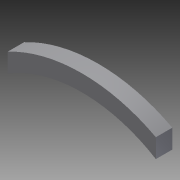
# Autodesk Inventor part: motor stay top
Saved by Autodesk Inventor 2012 (Build 160160000, 160)
## iProperties
Created: 2012-02-05
Part Number: motor stay top
Material: Default
Document SubType Name: Modeling
Designer: Antonella Wilby
Density: 1 g/cm^3
Author: Antonella Wilby
Autodesk Inventor part; units mm, degrees
ref_plane "YZ Plane" through (0, 0, 0) normal (1, 0, 0) x (0, 1, 0)
ref_plane "XZ Plane" through (0, 0, 0) normal (0, 1, 0) x (-1, 0, 0)
ref_plane "XY Plane" through (0, 0, 0) normal (0, 0, 1) x (1, 0, 0)
sketch "Sketch1" plane through (0, 0, 0) normal (0, 0, 1) x (1, 0, 0)
  line L0 (-75.565, 0) -> (75.565, 0) projected
  line L1 (0, -76.9938) -> (0, 84.1375) projected
  circle A0 centre (0, 0) radius 53.975 construction
  arc A1 (28.575, 46.7235) -> (-28.575, 46.7235) centre (0, 0) ccw
  arc A2 (28.575, 54.0275) -> (-28.575, 54.0275) centre (0, 0) ccw
  line L2 (-28.575, 46.7235) -> (-28.575, 54.0275)
  line L3 (28.575, 46.7235) -> (28.575, 54.0275)
  dimension "d0" = 107.95
  dimension "d1" = 0.7937
  dimension "d2" = 6.35
  dimension "d3" = 57.15
  constraints: 4 end point, 4 point on circle, 3 centre point, 2 parallel, 1 coincident, 1 other
  measures "d0" diameter of A0
  measures "d1" radial gap between concentric circles of A1 A0
  measures "d2" radial gap between concentric circles of A2 A1
  measures "d3" distance between parallel lines of L2 L3
extrude "Extrusion1" add sketch "Sketch1" along normal blind 6.35
body "Solid1"
